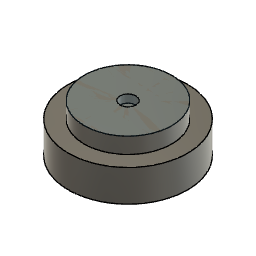
Braço Robótico v2 (Autodesk Fusion 360 archive; units mm, degrees)
design "Base do meio"
Autodesk Fusion 360 part; units mm, degrees
sketch "Sketch1" plane through (0, 0, 0) normal (0, 1, 0) x (1, 0, 0)
  circle A0 centre (0, 0) radius 75
  dimension "d1" = 150
  constraint coincident A0.centre origin
  measures "d1" diameter of A0
extrude "Extrude1" add sketch "Sketch1" along normal blind 40 makes body 1
sketch "Sketch2" plane through (0, 40, 0) normal (0, 1, 0) x (-1, 0, 0)
  circle A0 centre (0, 0) radius 75
  circle A1 centre (0, 0) radius 55
  dimension "d4" = 110
  constraint coincident A0.centre A1.centre
  measures "d4" diameter of A1
extrude "Extrude2" add sketch "Sketch2" along normal blind 20 contours A1 bodies 1
sketch "Sketch3" plane through (0, 60, 0) normal (0, 1, 0) x (-1, 0, 0)
  circle A0 centre (0, 0) radius 55
sketch "Sketch4" plane through (0, 60, 0) normal (0, 1, 0) x (-1, 0, 0)
  circle A0 centre (0, 0) radius 10
  dimension "d7" = 20
  constraint coincident A0.centre origin
  measures "d7" diameter of A0
extrude "Extrude3" cut sketch "Sketch4" against normal blind 10 bodies 1
sketch "Sketch6" plane through (0, 0, 0) normal (0, -1, 0) x (1, 0, 0)
  circle A0 centre (0, 0) radius 75
  circle A1 centre (0, 0) radius 12.5
  dimension "d10" = 25
  constraint concentric A0 A1
  measures "d10" diameter of A1
extrude "Extrude4" cut sketch "Sketch6" against normal blind 30 contours A1 bodies 1
copy_body "Body->Comp1" bodies 1 removing the originals makes body 2 in component "Component"
component "Component" placed x (1, 0, 0) y (0, 1, 0) z (0, 0, 1) at (0, 0, 0)

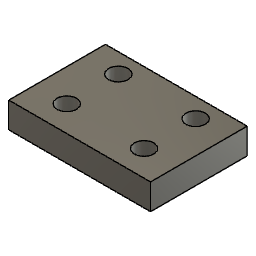
design "braçadeira"
Autodesk Fusion 360 part; units mm, degrees
sketch "Sketch1" plane through (0, 0, 0) normal (0, 1, 0) x (1, 0, 0)
  line L0 (0, 0) -> (22, 0)
  line L1 (22, 0) -> (22, -15)
  line L2 (22, -15) -> (0, -15)
  line L3 (0, -15) -> (0, 0)
  circle A0 centre (17, -11) radius 1.5
  line L4 (0, -15) -> (0, -14.748)
  circle A1 centre (5, -3) radius 1.5
  circle A2 centre (17, -3) radius 1.5
  circle A3 centre (5, -11) radius 1.5
  dimension "d11" = 3
  dimension "d18" = 3
  dimension "d21" = 3
  dimension "d24" = 3
  constraint horizontal L0
  constraint vertical L1
  constraint horizontal L2
  constraint vertical L3
  constraint coincident L0.start L3.end
  constraint coincident L3 L4.end
  measures "d11" diameter of A0
  measures "d18" diameter of A1
  measures "d21" diameter of A2
  measures "d24" diameter of A3
extrude "Extrude1" add sketch "Sketch1" along normal blind 4 makes body 1
copy_body "Body->Comp1" bodies 1 removing the originals makes body 2 in component "Component'"
component "Component'" placed x (1, 0, 0) y (0, 1, 0) z (0, 0, 1) at (0, 0, 0)

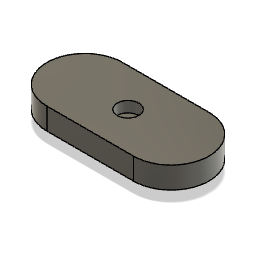
design "Base do meio"
Autodesk Fusion 360 part; units mm, degrees
sketch "Sketch1" plane through (0, 0, 0) normal (0, 1, 0) x (1, 0, 0)
  line L0 (75, -35) -> (-75, -35)
  line L1 (-75, -35) -> (-75, 35)
  line L2 (-75, 35) -> (75, 35)
  line L3 (75, 35) -> (75, -35)
  line L4 (75, -35) -> (-75, 35) construction
  line L5 (-75, -35) -> (75, 35) construction
  dimension "d1" = 150
  dimension "d2" = 70
  constraint horizontal L0
  constraint perpendicular L0 L1
  constraint parallel L0 L2
  constraint parallel L1 L3
  constraint coincident L4 origin
  constraint coincident L5 origin
  measures "d1" distance of L1.end L2.end
  measures "d2" distance of L0.end L1.end
extrude "Extrude1" add sketch "Sketch1" along normal blind 20 makes body 1
fillet "Fillet1" radius 35 4 edges at (-75, 10, 35) (75, 10, 35) (75, 10, -35) (-75, 10, -35) on bodies 1
sketch "Sketch2" plane through (0, 0, 0) normal (0, -1, 0) x (1, 0, 0)
  arc A0 (-40, 35) -> (-40, -35) centre (-40, 0) ccw
  line L0 (-40, -35) -> (40, -35)
  arc A1 (40, -35) -> (40, 35) centre (40, 0) ccw
  line L1 (40, 35) -> (-40, 35)
  circle A2 centre (0, 0) radius 10
  dimension "d7" = 20
  constraint coincident A2.centre origin
  measures "d7" diameter of A2
extrude "Extrude2" add sketch "Sketch2" along normal blind 10 contours A2 bodies 1
sketch "Sketch3" plane through (0, 20, 0) normal (0, 1, 0) x (-1, 0, 0)
  arc A0 (40, -35) -> (40, 35) centre (40, 0) ccw
  line L0 (40, 35) -> (-40, 35)
  arc A1 (-40, 35) -> (-40, -35) centre (-40, 0) ccw
  line L1 (-40, -35) -> (40, -35)
  circle A2 centre (0, 0) radius 10
  dimension "d10" = 20
  constraint coincident A2.centre origin
  measures "d10" diameter of A2
extrude "Extrude3" cut sketch "Sketch3" against normal blind 10 contours A2 bodies 1
copy_body "Body->Comp1" bodies 1 removing the originals makes body 2 in component "Component"
component "Component" placed x (1, 0, 0) y (0, 1, 0) z (0, 0, 1) at (0, 0, 0)

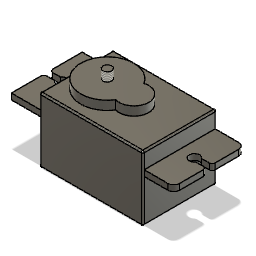
design "ServoMotor representação"
Autodesk Fusion 360 part; units mm, degrees
sketch "Sketch1" plane through (0, 0, 0) normal (0, 1, 0) x (1, 0, 0)
  line L0 (0, 0) -> (35, 0)
  line L1 (35, 0) -> (35, -25)
  line L2 (35, -25) -> (0, -25)
  line L3 (0, -25) -> (0, 0)
  dimension "d1" = 35
  dimension "d2" = 25
  constraint horizontal L0
  constraint vertical L1
  constraint horizontal L2
  constraint vertical L3
  constraint coincident L0.start L3.end
  measures "d1" distance of L0.start L0.end
  measures "d2" distance of L0.start L2.end
extrude "Extrude1" add sketch "Sketch1" along normal blind 22 makes body 1
fillet "Fillet1" radius 0.5 12 edges at (35, 22, 12.5) (17.5, 22, 25) (0, 22, 12.5) (17.5, 22, 0) (17.5, 0, 25) (35, 0, 12.5) (35, 11, 0) (35, 11, 25) (17.5, 0, 0) (0, 11, 0) (0, 11, 25) (0, 0, 12.5) on bodies 1
sketch "Sketch2" plane through (0, 22, 0) normal (0, 1, 0) x (-1, 0, 0)
  line L0 (-34.5, 0.5) -> (-0.5, 0.5)
  line L1 (-0.5, 0.5) -> (-0.5, 24.5)
  line L2 (-0.5, 24.5) -> (-34.5, 24.5)
  line L3 (-34.5, 24.5) -> (-34.5, 0.5)
  arc A0 (-18.1111, 17.3032) -> (-18.1111, 7.6968) centre (-19.5, 12.5) ccw
  arc A1 (-18.1111, 7.6968) -> (-18.1111, 17.3032) centre (-10.5, 12.5) ccw
  dimension "d8" = 18
  measures "d8" diameter of A1
extrude "Extrude2" add sketch "Sketch2" along normal blind 3 contours A0 A1 bodies 1
sketch "Sketch3" plane through (0, 25, 0) normal (0, 1, 0) x (-1, 0, 0)
  arc A0 (-18.1111, 7.6968) -> (-18.1111, 17.3032) centre (-10.5, 12.5) ccw
  arc A1 (-18.1111, 17.3032) -> (-18.1111, 7.6968) centre (-19.5, 12.5) ccw
  circle A2 centre (-10.5, 12.5) radius 1.5
  dimension "d20" = 3
  constraint concentric A0 A2
  measures "d20" diameter of A2
extrude "Extrude3" add sketch "Sketch3" along normal blind 3 contours A2 bodies 1
thread "Thread1" "ISO Metric profile 3.0 M3x0.5 6g" major diameter 2.927 minor diameter 2.3555 pitch 0.5 angle 60 resizes the face on face at (9.0019, 27, 12.4252) on bodies 1
sketch "Sketch4" plane through (35, 0, 0) normal (1, 0, 0) x (0, 0, -1)
  line L0 (-24.5, 0.5) -> (-0.5, 0.5)
  line L1 (-0.5, 0.5) -> (-0.5, 21.5)
  line L2 (-0.5, 21.5) -> (-24.5, 21.5)
  line L3 (-24.5, 21.5) -> (-24.5, 0.5)
  line L4 (-12.5, 21.5) -> (-12.5, 16.5)
  line L5 (-12.5, 16.5) -> (-24.5, 16.5)
  line L6 (-12.5, 16.5) -> (-0.5, 16.5)
  line L7 (-24.5, 16.5) -> (-24.5, 14.5)
  line L8 (-24.5, 14.5) -> (-0.5, 14.5)
  line L9 (-0.5, 14.5) -> (-0.5, 16.5)
  dimension "d23" = 5
  dimension "d24" = 12
  dimension "d25" = 12
  dimension "d26" = 2
  dimension "d27" = 24
  constraint midpoint L2 L4.start
  constraint perpendicular L2 L4
  constraint perpendicular L3 L5
  constraint perpendicular L4 L6
  constraint perpendicular L5 L7
  constraint perpendicular L7 L8
  measures "d23" distance of L4.start L4.end
  measures "d24" distance of L4.end L5.end
  measures "d25" distance of L4.end L6.end
  measures "d26" distance of L5.end L7.end
  measures "d27" distance of L7.end L8.end
extrude "Extrude4" add sketch "Sketch4" along normal blind 10 contours L1 L3 L5 L6 L7 L8 L9 bodies 1
fillet "Fillet2" radius 2 2 edges at (45, 15.5, 24.5) (45, 15.5, 0.5) on bodies 1
sketch "Sketch5" plane through (0, 16.5, 0) normal (0, 1, 0) x (-1, 0, 0)
  arc A0 (-45, 2.5) -> (-43, 0.5) centre (-43, 2.5) ccw
  line L0 (-43, 0.5) -> (-35, 0.5)
  line L1 (-35, 0.5) -> (-35, 24.5)
  line L2 (-35, 24.5) -> (-43, 24.5)
  arc A1 (-43, 24.5) -> (-45, 22.5) centre (-43, 22.5) ccw
  line L3 (-45, 22.5) -> (-45, 2.5)
  line L4 (-45, 12.5) -> (-45, 11.5)
  line L5 (-45, 12.5) -> (-45, 13.5)
  line L6 (-45, 13.5) -> (-41.4361, 13.5)
  line L7 (-45, 11.5) -> (-41.4361, 11.5)
  arc A2 (-41.4361, 11.5) -> (-41.4361, 13.5) centre (-40, 12.5) ccw
  dimension "d32" = 5
  dimension "d33" = 3.5
  dimension "d34" = 1
  dimension "d35" = 1
  constraint midpoint L3 L4.start
  constraint coincident L3 L5.end
  constraint perpendicular L5 L6
  constraint perpendicular L3 L7
  measures "d32" distance of L4.start A2.centre
  measures "d33" diameter of A2
  measures "d34" distance of L4.start L4.end
  measures "d35" distance of L4.start L5.end
extrude "Extrude5" cut sketch "Sketch5" against normal blind 6.2 contours L3 L4 L5 L6 L7 A2 bodies 1
fillet "Fillet3" radius 1 2 edges at (45, 15.5, 11.5) (45, 15.5, 13.5) on bodies 1
sketch "Sketch6" plane through (0, 0, 0) normal (-1, 0, 0) x (0, 0, 1)
  line L0 (24.5, 0.5) -> (24.5, 21.5)
  line L1 (24.5, 21.5) -> (0.5, 21.5)
  line L2 (0.5, 21.5) -> (0.5, 0.5)
  line L3 (0.5, 0.5) -> (24.5, 0.5)
  line L4 (0.5, 16.5) -> (24.5, 16.5)
  line L5 (24.5, 16.5) -> (24.5, 14.5)
  line L6 (24.5, 14.5) -> (0.5, 14.5)
  line L7 (0.5, 14.5) -> (0.5, 16.5)
  dimension "d40" = 5
  dimension "d41" = 24
  dimension "d42" = 2
  constraint horizontal L4
  constraint vertical L5
  constraint horizontal L6
  constraint vertical L7
  measures "d40" distance of L1.end L4.start
  measures "d41" distance of L4.start L4.end
  measures "d42" distance of L4.start L6.end
extrude "Extrude6" add sketch "Sketch6" along normal blind 10 contours L0 L2 L4 L5 L6 L7 bodies 1
sketch "Sketch7" plane through (0, 16.5, 0) normal (0, 1, 0) x (-1, 0, 0)
  line L0 (0, 24.5) -> (0, 0.5)
  line L1 (0, 0.5) -> (10, 0.5)
  line L2 (10, 0.5) -> (10, 24.5)
  line L3 (10, 24.5) -> (0, 24.5)
  line L4 (0, 12.5) -> (5, 12.5)
  line L5 (10, 12.5) -> (10, 11.5)
  line L6 (10, 12.5) -> (10, 13.5)
  line L7 (10, 11.5) -> (6.4361, 11.5)
  line L8 (10, 13.5) -> (6.4361, 13.5)
  arc A0 (6.4361, 13.5) -> (6.4361, 11.5) centre (5, 12.5) ccw
  dimension "d45" = 5
  dimension "d46" = 3.5
  dimension "d47" = 1
  dimension "d48" = 1
  constraint midpoint L0 L4.start
  constraint perpendicular L0 L4
  constraint coincident L4.end A0.centre
  constraint midpoint L2 L5.start
  constraint perpendicular L5 L7
  constraint perpendicular L6 L8
  measures "d45" distance of L4.start L4.end
  measures "d46" diameter of A0
  measures "d47" distance of L5.start L5.end
  measures "d48" distance of L5.start L6.end
extrude "Extrude7" cut sketch "Sketch7" against normal blind 6.5 contours L2 L5 L6 L7 L8 A0 bodies 1
fillet "Fillet4" radius 1 2 edges at (-10, 15.5, 13.5) (-10, 15.5, 11.5) on bodies 1
copy_body "Body->Comp1" bodies 1 removing the originals makes body 2 in component "Component'"
component "Component'" placed x (1, 0, 0) y (0, 1, 0) z (0, 0, 1) at (0, 0, 0)

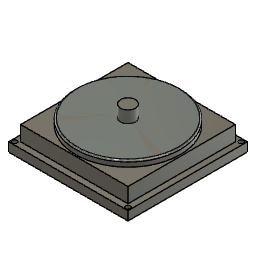
design "Peça 1"
Autodesk Fusion 360 part; units mm, degrees
sketch "Sketch1" plane through (0, 0, 0) normal (0, 1, 0) x (1, 0, 0)
  line L0 (90, -90) -> (-90, -90)
  line L1 (-90, -90) -> (-90, 90)
  line L2 (-90, 90) -> (90, 90)
  line L3 (90, 90) -> (90, -90)
  line L4 (90, -90) -> (-90, 90) construction
  line L5 (-90, -90) -> (90, 90) construction
  line L6 (100, -100) -> (-100, -100)
  line L7 (-100, -100) -> (-100, 100)
  line L8 (-100, 100) -> (100, 100)
  line L9 (100, 100) -> (100, -100)
  line L10 (100, -100) -> (-100, 100) construction
  line L11 (-100, -100) -> (100, 100) construction
  line L12 (-100, 100) -> (-90, 90)
  line L13 (100, 100) -> (90, 90)
  line L14 (90, -90) -> (100, -100)
  line L15 (-90, -90) -> (-100, -100)
  circle A0 centre (-95, -95) radius 4
  circle A1 centre (-95, 95) radius 4
  circle A2 centre (95, 95) radius 4
  circle A3 centre (95, -95) radius 4
  dimension "d3" = 180
  dimension "d4" = 180
  dimension "d5" = 200
  dimension "d6" = 200
  dimension "d7" = 8
  dimension "d8" = 8
  dimension "d9" = 8
  dimension "d10" = 8
  constraint horizontal L0
  constraint perpendicular L0 L1
  constraint parallel L0 L2
  constraint parallel L1 L3
  constraint coincident L4 origin
  constraint coincident L5 origin
  constraint horizontal L6
  constraint perpendicular L6 L7
  constraint parallel L6 L8
  constraint parallel L7 L9
  constraint coincident L10 origin
  constraint coincident L11 origin
  constraint midpoint L15 A0.centre
  constraint midpoint L12 A1.centre
  constraint midpoint L13 A2.centre
  constraint midpoint L14 A3.centre
  measures "d3" distance of L1.end L2.end
  measures "d4" distance of L0.end L1.end
  measures "d5" distance of L7.end L8.end
  measures "d6" distance of L6.end L7.end
  measures "d7" diameter of A0
  measures "d8" diameter of A1
  measures "d9" diameter of A2
  measures "d10" diameter of A3
extrude "Extrude1" add sketch "Sketch1" along normal blind 40 contours L0 L1 L2 L3
extrude "Extrude2" add sketch "Sketch1" along normal blind 15 contours L0 L6 L14 L15 A0 A3 | L3 L9 L13 L14 A2 A3 | L1 L7 L12 L15 A0 A1 | L2 L8 L12 L13 A1 A2
sketch "Sketch2" plane through (0, 40, 0) normal (0, 1, 0) x (-1, 0, 0)
  line L0 (-90, -90) -> (90, -90)
  line L1 (90, -90) -> (90, 90)
  line L2 (90, 90) -> (-90, 90)
  line L3 (-90, 90) -> (-90, -90)
  circle A0 centre (0, 0) radius 87.5
  circle A1 centre (0, 0) radius 12.5
  dimension "d15" = 175
  dimension "d16" = 25
  constraint coincident A0.centre A1.centre
  constraint concentric A0 A1
  measures "d15" diameter of A0
  measures "d16" diameter of A1
extrude "Extrude3" add sketch "Sketch2" along normal blind 30 contours A1
extrude "Extrude4" add sketch "Sketch2" along normal blind 10 contours A0
fillet "Fillet1" radius 2.5 1 edges at (81.5786, 50, -31.6414)
sketch "Sketch3" plane through (0, 50, 0) normal (0, 1, 0) x (-1, 0, 0)
  circle A0 centre (0, 0) radius 12.5
  circle A1 centre (0, 0) radius 85

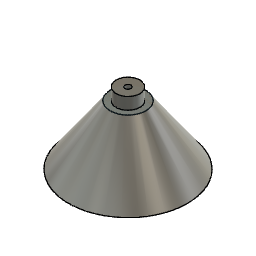
design "conexão"
Autodesk Fusion 360 part; units mm, degrees
sketch "Sketch1" plane through (0, 0, 0) normal (0, 1, 0) x (1, 0, 0)
  circle A0 centre (0, 0) radius 50
  dimension "d1" = 100
  constraint coincident A0.centre origin
  measures "d1" diameter of A0
extrude "Extrude1" add sketch "Sketch1" along normal blind 50 draft -35 makes body 1
sketch "Sketch2" plane through (0, 50, 0) normal (0, 1, 0) x (-1, 0, 0)
  circle A0 centre (0, 0) radius 14.9896
sketch "Sketch3" plane through (0, 50, 0) normal (0, 1, 0) x (-1, 0, 0)
  circle A0 centre (0, 0) radius 10
  dimension "d5" = 20
  constraint coincident A0.centre origin
  measures "d5" diameter of A0
extrude "Extrude2" add sketch "Sketch3" along normal blind 10 bodies 1
sketch "Sketch4" plane through (0, 60, 0) normal (0, 1, 0) x (-1, 0, 0)
  circle A0 centre (0, 0) radius 10
  circle A1 centre (0, 0) radius 2.4995
  dimension "d8" = 4.999
  constraint concentric A0 A1
  measures "d8" diameter of A1
extrude "Extrude3" cut sketch "Sketch4" against normal blind 5 contours A1 bodies 1
copy_body "Body->Comp1" bodies 1 removing the originals makes body 2 in component "Component'"
component "Component'" placed x (1, 0, 0) y (0, 1, 0) z (0, 0, 1) at (0, 0, 0)

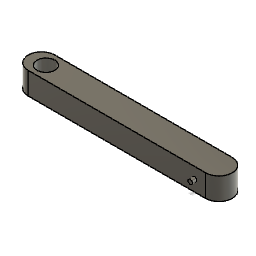
design "Segunda parte Braço"
Autodesk Fusion 360 part; units mm, degrees
sketch "Sketch1" plane through (0, 0, 0) normal (0, 1, 0) x (1, 0, 0)
  line L0 (100, -15) -> (-100, -15)
  line L1 (-100, -15) -> (-100, 15)
  line L2 (-100, 15) -> (100, 15)
  line L3 (100, 15) -> (100, -15)
  line L4 (100, -15) -> (-100, 15) construction
  line L5 (-100, -15) -> (100, 15) construction
  arc A0 (-95.599, 14.3399) -> (-95.599, -14.3399) centre (-100, 0) ccw
  arc A1 (95.599, -14.3399) -> (95.599, 14.3399) centre (100, 0) ccw
  dimension "d1" = 200
  dimension "d2" = 30
  constraint horizontal L0
  constraint perpendicular L0 L1
  constraint parallel L0 L2
  constraint parallel L1 L3
  constraint coincident L4 origin
  constraint coincident L5 origin
  constraint midpoint L3 A1.centre
  constraint coincident L2.end A1
  constraint midpoint L1 A0.centre
  constraint coincident L1.end A0
  constraint coincident L5 A0.end
  constraint coincident L4 A0.start
  constraint coincident L5 A1.end
  constraint coincident L4 A1.start
  measures "d1" distance of L1.end L2.end
  measures "d2" distance of L0.end L1.end
extrude "Extrude1" add sketch "Sketch1" along normal blind 25 makes body 1
sketch "Sketch2" plane through (0, 25, 0) normal (0, 1, 0) x (-1, 0, 0)
  arc A0 (100, -15) -> (100, 15) centre (100, 0) ccw
  line L0 (100, 15) -> (-100, 15)
  arc A1 (-100, 15) -> (-100, -15) centre (-100, 0) ccw
  line L1 (-100, -15) -> (100, -15)
  circle A2 centre (95, 0) radius 10
  dimension "d6" = 20
  measures "d6" diameter of A2
extrude "Extrude2" cut sketch "Sketch2" against normal blind 70 contours A2 bodies 1
sketch "Sketch3" plane through (0, 0, -15) normal (0, 0, -1) x (-1, 0, 0)
  line L0 (-100, 0) -> (100, 0)
  line L1 (100, 0) -> (100, 25)
  line L2 (100, 25) -> (-100, 25)
  line L3 (-100, 25) -> (-100, 0)
  line L4 (-85, 15.675) -> (-85, 15.5847)
  line L5 (-86.7208, 15.1734) -> (-85, 15.1734)
  line L6 (-83.2872, 15.1734) -> (-83.2758, 15.1734)
  line L7 (-85, 15.1734) -> (-83.2758, 15.1734)
  arc A0 (-86.7128, 15.1734) -> (-83.2872, 15.1734) centre (-85, 12.5) ccw
  dimension "d11" = 6.35
  dimension "d18" = 3.445
  constraint perpendicular L4 L5
  constraint collinear L5 L6
  constraint parallel L6 L7
  constraint coincident L5 A0.start
  measures "d11" diameter of A0
  measures "d18" distance of L5.start L6.end
extrude "Extrude3" cut sketch "Sketch3" against normal blind 14.986 contours L5 L7 A0 bodies 1
sketch "Sketch4" plane through (0, 0, 15) normal (0, 0, 1) x (1, 0, 0)
  line L0 (-100, 0) -> (100, 0)
  line L1 (100, 0) -> (100, 25)
  line L2 (100, 25) -> (-100, 25)
  line L3 (-100, 25) -> (-100, 0)
  circle A0 centre (87.5, 12.5) radius 2.4995
  dimension "d15" = 4.999
  measures "d15" diameter of A0
extrude "Extrude4" add sketch "Sketch4" along normal blind 5 contours A0 bodies 1
copy_body "Body->Comp1" bodies 1 removing the originals makes body 2 in component "Component'"
component "Component'" placed x (1, 0, 0) y (0, 1, 0) z (0, 0, 1) at (0, 0, 0)

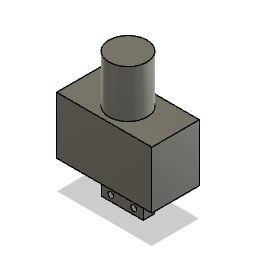
design "Base da garra"
Autodesk Fusion 360 part; units mm, degrees
sketch "Sketch1" plane through (0, 0, 0) normal (0, 1, 0) x (1, 0, 0)
  line L0 (25, -12.5) -> (-25, -12.5)
  line L1 (-25, -12.5) -> (-25, 12.5)
  line L2 (-25, 12.5) -> (25, 12.5)
  line L3 (25, 12.5) -> (25, -12.5)
  line L4 (25, -12.5) -> (-25, 12.5) construction
  line L5 (-25, -12.5) -> (25, 12.5) construction
  dimension "d1" = 50
  dimension "d2" = 25
  constraint horizontal L0
  constraint perpendicular L0 L1
  constraint parallel L0 L2
  constraint parallel L1 L3
  constraint coincident L4 origin
  constraint coincident L5 origin
  measures "d1" distance of L1.end L2.end
  measures "d2" distance of L0.end L1.end
extrude "Extrude1" add sketch "Sketch1" along normal blind 30 makes body 1
sketch "Sketch2" plane through (0, 30, 0) normal (0, 1, 0) x (-1, 0, 0)
  line L0 (-25, -12.5) -> (25, -12.5)
  line L1 (25, -12.5) -> (25, 12.5)
  line L2 (25, 12.5) -> (-25, 12.5)
  line L3 (-25, 12.5) -> (-25, -12.5)
  circle A0 centre (0, 0) radius 10
  dimension "d5" = 20
  constraint coincident A0.centre origin
  measures "d5" diameter of A0
extrude "Extrude2" add sketch "Sketch2" along normal blind 25 contours A0 bodies 1
sketch "Sketch3" plane through (0, 0, 0) normal (0, -1, 0) x (1, 0, 0)
  line L0 (-25, -12.5) -> (25, -12.5)
  line L1 (25, -12.5) -> (25, 12.5)
  line L2 (25, 12.5) -> (-25, 12.5)
  line L3 (-25, 12.5) -> (-25, -12.5)
  line L4 (11, -3) -> (-11, -3)
  line L5 (-11, -3) -> (-11, 3)
  line L6 (-11, 3) -> (11, 3)
  line L7 (11, 3) -> (11, -3)
  line L8 (11, -3) -> (-11, 3) construction
  line L9 (-11, -3) -> (11, 3) construction
  dimension "d8" = 22
  dimension "d9" = 6
  constraint horizontal L4
  constraint perpendicular L4 L5
  constraint parallel L4 L6
  constraint parallel L5 L7
  constraint coincident L8 origin
  constraint coincident L9 origin
  measures "d8" distance of L5.end L6.end
  measures "d9" distance of L4.end L5.end
extrude "Extrude4" add sketch "Sketch3" along normal blind 10 contours L4 L5 L6 L7 bodies 1
sketch "Sketch4" plane through (0, 0, 3) normal (0, 0, 1) x (1, 0, 0)
  line L0 (11, 0) -> (-11, 0)
  line L1 (-11, 0) -> (-11, -10)
  line L2 (-11, -10) -> (11, -10)
  line L3 (11, -10) -> (11, 0)
  circle A0 centre (-6, -7) radius 1.5
  circle A1 centre (6, -7) radius 1.5
  dimension "d16" = 3
  dimension "d19" = 3
  measures "d16" diameter of A0
  measures "d19" diameter of A1
extrude "Extrude5" cut sketch "Sketch4" against normal blind 15 contours A0 | A1 bodies 1
extrude "Extrude3" add sketch "Sketch3" along normal blind 15 contours L4 L5 L6 L7 bodies 1
sketch "Sketch5" plane through (0, 0, 3) normal (0, 0, 1) x (1, 0, 0)
  line L0 (11, 0) -> (-11, 0)
  line L1 (-11, 0) -> (-11, -15)
  line L2 (-11, -15) -> (11, -15)
  line L3 (11, -15) -> (11, 0)
  circle A0 centre (-6, -12) radius 1.5
  circle A1 centre (6, -12) radius 1.5
  dimension "d26" = 3
  dimension "d27" = 3
  measures "d26" diameter of A0
  measures "d27" diameter of A1
extrude "Extrude6" cut sketch "Sketch5" against normal blind 21 contours A0 | A1 bodies 1
copy_body "Body->Comp2" bodies 1 removing the originals makes body 2 in component "Component"
component "Component" placed x (1, 0, 0) y (0, 1, 0) z (0, 0, 1) at (0, 0, 0)
